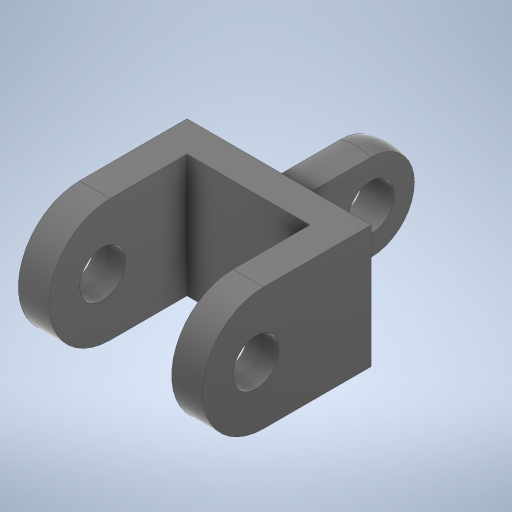
# Autodesk Inventor part: Claw Palm
Saved by Autodesk Inventor 2024 (Build 280153000, 153)
## iProperties
Created: 2023-06-06
Part Number: Claw Palm
Material: Generic
Document SubType Name: Modeling
Designer: vilas
Density: 1 g/cm^3
Appearance: Default
Author: vilas
Autodesk Inventor part; units mm, degrees
ref_plane "YZ Plane" through (0, 0, 0) normal (1, 0, 0) x (0, 1, 0)
ref_plane "XZ Plane" through (0, 0, 0) normal (0, 1, 0) x (-1, 0, 0)
ref_plane "XY Plane" through (0, 0, 0) normal (0, 0, 1) x (1, 0, 0)
sketch "Sketch1" plane through (0, 0, 0) normal (0, 0, 1) x (1, 0, 0)
  line L0 (2.5, -7.5) -> (-2.5, -7.5)
  line L1 (-2.5, -7.5) -> (-2.5, 7.5)
  line L2 (-2.5, 7.5) -> (2.5, 7.5) construction
  line L3 (2.5, 7.5) -> (2.5, -7.5)
  line L4 (2.5, -7.5) -> (-2.5, 7.5) construction
  line L5 (-2.5, -7.5) -> (2.5, 7.5) construction
  arc A0 (2.5, 7.0711) -> (-2.5, 7.0711) centre (0, 0) ccw
  arc A1 (-2.5, -7.0711) -> (2.5, -7.0711) centre (0, 0) ccw
  dimension "d0" = 5
  dimension "d1" = 15
  dimension "d2" = 7.5
  dimension "d3" = 7.5
  constraints: 12 end point, 4 point on circle, 4 point on line, 2 centre point, 2 coincident, 2 midpoint, 2 parallel, 1 horizontal, 1 perpendicular
  measures "d0" distance of L1.end L2.end
  measures "d1" distance between parallel lines of L0 L2
  measures "d2" radius of A0
  measures "d3" radius of A1
extrude "Extrusion1" add sketch "Sketch1" along normal blind 20 contours A1 L1 A0 L3
sketch "Sketch2" plane through (0, 0, 0) normal (1, 0, 0) x (0, 1, 0)
  line L0 (7.0711, 20) -> (-7.0711, 20) projected
  line L1 (0, 20) -> (0, 7.5) construction
  circle A0 centre (0, 7.5) radius 3.75
  point P0 (0, 0)
  dimension "d6" = 12.5
  dimension "d7" = 7.5
  constraints: 2 end point, 1 centre point, 1 coincident, 1 midpoint, 1 vertical
  measures "d6" distance of L1.start L1.end
  measures "d7" diameter of A0
extrude "Extrusion2" cut sketch "Sketch2" along normal through all both and the other way through all
fillet "Fillet1" radius 7.5 1 edges at (0, 7.5, 0)
sketch "Sketch3" plane through (0, 0, 20) normal (0, 0, 1) x (1, 0, 0)
  line L0 (-15, 10) -> (15, 10)
  line L1 (15, 10) -> (15, -10)
  line L2 (15, -10) -> (-15, -10)
  line L3 (-15, -10) -> (-15, 10)
  line L4 (-15, 10) -> (15, -10) construction
  line L5 (15, 10) -> (-15, -10) construction
  point P0 (0, 0)
  dimension "d11" = 30
  dimension "d12" = 20
  constraints: 12 end point, 2 midpoint, 2 parallel, 1 horizontal, 1 perpendicular
  measures "d11" distance of L1.end L2.end
  measures "d12" distance of L0.end L1.end
extrude "Extrusion3" add sketch "Sketch3" along normal blind 5
sketch "Sketch4" plane through (0, 0, 25) normal (0, 0, 1) x (1, 0, 0)
  line L0 (-15, 10) -> (-15, -10) projected
  line L1 (-15, -10) -> (15, -10) projected
  line L2 (-15, 10) -> (-10, 10)
  line L3 (-10, 10) -> (-10, -10)
  line L4 (-10, -10) -> (-15, -10)
  line L5 (-15, -10) -> (-15, 10)
  line L6 (15, -10) -> (15, 10) projected
  line L7 (15, -10) -> (10, -10)
  line L8 (10, -10) -> (10, 10)
  line L9 (10, 10) -> (15, 10)
  line L10 (15, 10) -> (15, -10)
  point P0 (0, 0)
  dimension "d15" = 5
  dimension "d16" = 5
  constraints: 16 end point, 4 parallel, 2 horizontal, 2 perpendicular, 2 point on line
  measures "d15" distance of L3.end L4.end
  measures "d16" distance of L8.end L9.end
extrude "Extrusion4" add sketch "Sketch4" along normal blind 22.5
sketch "Sketch5" plane through (0, 0, 0) normal (1, 0, 0) x (0, 1, 0)
  line L0 (-10, 25) -> (10, 25) projected
  line L1 (0, 25) -> (0, 38.75) construction
  circle A0 centre (0, 38.75) radius 3.75
  point P0 (0, 0)
  dimension "d19" = 13.75
  dimension "d20" = 7.5
  constraints: 2 end point, 1 centre point, 1 coincident, 1 midpoint, 1 vertical
  measures "d19" distance of L1.start L1.end
  measures "d20" diameter of A0
extrude "Extrusion5" cut sketch "Sketch5" along normal through all both and the other way through all
fillet "Fillet2" radius 10 4 edges at (-12.5, 10, 47.5) (-12.5, -10, 47.5) (12.5, 10, 47.5) (12.5, -10, 47.5)
body "Solid1"
